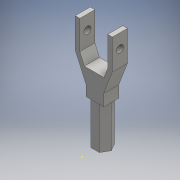
# Autodesk Inventor part: Test de pincev2
Saved by Autodesk Inventor 2016 (Build 200138000, 138)
## iProperties
Created: 2016-04-01
Part Number: Test de pincev2
Material: Generic
Document SubType Name: Modeling
Designer: Thetheos
Density: 1 g/cm^3
Appearance: Default
Author: Thetheos
Autodesk Inventor part; units mm, degrees
ref_plane "YZ Plane" through (0, 0, 0) normal (1, 0, 0) x (0, 1, 0)
ref_plane "XZ Plane" through (0, 0, 0) normal (0, 1, 0) x (-1, 0, 0)
ref_plane "XY Plane" through (0, 0, 0) normal (0, 0, 1) x (1, 0, 0)
sketch "Sketch1" plane through (0, 0, 0) normal (0, 0, 1) x (1, 0, 0)
  line L0 (9.75, 13) -> (7.875, 9.7524)
  line L1 (7.875, 9.7524) -> (4.125, 9.7524)
  line L2 (4.125, 9.7524) -> (2.25, 13)
  line L3 (2.25, 13) -> (4.125, 16.2476)
  line L4 (4.125, 16.2476) -> (7.875, 16.2476)
  line L5 (7.875, 16.2476) -> (9.75, 13)
  point P0 (0, 0)
  point P1 (6, 13)
  dimension "d0" = 7.5
  constraints: 12 end point, 13 other
  measures "d0" distance of L0.start L2.end
extrude "Extrusion1" add sketch "Sketch1" along normal blind 18
sketch "Sketch2" plane through (4.125, 16.2476, 0) normal (0, 1, 0) x (1, 0, 0)
  line L0 (3.75, -18) -> (5.625, -18) projected
  line L1 (3.75, -18) -> (0, -18) projected
  line L2 (0, -18) -> (-6.6597, -33.0128)
  line L3 (-1.875, 0) -> (-1.875, -18) projected
  line L4 (-6.6597, -45.8247) -> (-6.6597, -33.0128)
  line L5 (3.75, -18) -> (1.875, -18)
  line L6 (9.3403, -45.8668) -> (9.3403, -32.8539)
  line L7 (9.3403, -32.8539) -> (3.75, -18)
  line L8 (9.3403, -45.8668) -> (7.3403, -45.8668)
  line L9 (7.3403, -45.8668) -> (7.3403, -33.2178)
  line L10 (-6.6597, -45.8247) -> (-4.6597, -45.8247)
  line L11 (-4.6597, -45.8247) -> (-4.6597, -33.4364)
  line L12 (2.1735, -18.0436) -> (2.158, -18)
  line L13 (1.875, -29) -> (5.7529, -29)
  line L14 (-2.6917, -29) -> (1.875, -29)
  line L15 (-4.6597, -33.4364) -> (-2.6917, -29)
  line L16 (5.7529, -29) -> (7.3403, -33.2178)
  line L17 (1.875, -18) -> (1.875, -45.8247)
  point P0 (-4.125, 0)
  dimension "d12" = 2
  dimension "d13" = 2
  dimension "d16" = 27.8247
  dimension "d17" = 11
  dimension "d21" = 12
  dimension "d31" = 2
  dimension "d32" = 2
  constraints: 30 end point, 3 parallel, 3 vertical, 2 horizontal, 2 perpendicular, 2 point on line, 1 collinear, 1 midpoint
  measures "d12" distance of L6.start L8.end
  measures "d13" distance of L4.start L10.end
  measures "d16" distance between parallel lines of L10 L1
  measures "d17" distance of L5.end L13.start
  measures "d21" distance between parallel lines of L9 L11
  measures "d31" distance between parallel lines of L2 L15
  measures "d32" distance between parallel lines of L7 L16
extrude "Extrusion2" add sketch "Sketch2" against normal blind 6.5
sketch "Sketch3" plane through (-2.5347, 9.7476, 33.0128) normal (-0.9141, 0, -0.4055) x (-0.4055, 0, 0.9141)
  point P0 (-31.2047, -9.7476)
sketch "Sketch5" plane through (4.125, 16.2476, 0) normal (0, 1, 0) x (1, 0, 0)
  line L0 (-1.875, -18) -> (0, -18) projected
  line L1 (-1.875, -18) -> (-1.875, -22.2268)
  line L2 (0, -18) -> (-6.6597, -33.0128) projected
  line L3 (3.75, -18) -> (5.625, -18) projected
  line L4 (5.625, -18) -> (5.625, -22.982)
  line L5 (9.3403, -32.8539) -> (3.75, -18) projected
  point P0 (-4.125, 0)
  constraints: 4 end point, 2 perpendicular, 2 point on line, 1 parallel, 1 vertical
extrude "Extrusion3" add sketch "Sketch5" against normal blind 6.5
sketch "Sketch6" plane through (13.4653, 16.2476, 45.8668) normal (1, 0, 0) x (0, 0, -1)
  line L0 (0, 0) -> (0, -3.25)
  line L1 (0, 0) -> (0, -6.5) projected
  line L2 (0, -3.25) -> (6, -3.25)
  circle A0 centre (6, -3.25) radius 1.5
  point P0 (45.8668, -16.2476)
  dimension "d27" = 6
  dimension "d28" = 3
  constraints: 4 end point, 1 centre point, 1 coincident, 1 midpoint
  measures "d27" distance of L0.end L2.end
  measures "d28" diameter of A0
extrude "Extrusion4" cut sketch "Sketch6" against normal through all
body "Solid1"
